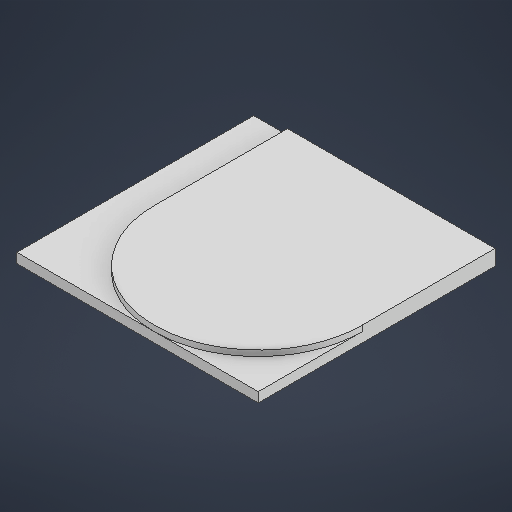
# Autodesk Inventor part: klapka
Saved by Autodesk Inventor 2026.1 (Build 301233020, 233B)
## iProperties
Created: 2025-08-31
Part Number: klapka
Material: Ogólny
Document SubType Name: Modeling
Designer: Paweł
Density: 1 g/cm^3
Appearance: Domyślna
Author: Paweł
Autodesk Inventor part; units mm, degrees
ref_plane "YZ Plane" through (0, 0, 0) normal (1, 0, 0) x (0, 1, 0)
ref_plane "XZ Plane" through (0, 0, 0) normal (0, 1, 0) x (-1, 0, 0)
ref_plane "XY Plane" through (0, 0, 0) normal (0, 0, 1) x (1, 0, 0)
sketch "Sketch1" plane through (0, 0, 0) normal (0, 0, 1) x (1, 0, 0)
  point P0 (0, 0)
sketch "Sketch2" plane through (0, 0, 0) normal (0, 1, 0) x (-1, 0, 0)
  line L0 (11.1114, 10.1278) -> (-7.2886, 10.1278)
  line L1 (-7.2886, 10.1278) -> (-7.2886, -10.8722)
  line L2 (-7.2886, -10.8722) -> (11.1114, -10.8722)
  line L3 (11.1114, -10.8722) -> (11.1114, 10.1278)
  point P0 (0, 0)
  dimension "d0" = 21
  dimension "d1" = 18.4
  constraints: 8 end point, 2 parallel, 1 horizontal, 1 perpendicular
  measures "d0" distance of L2.end L0.start
  measures "d1" distance of L0.start L0.end
extrude "Extrusion1" add sketch "Sketch2" along normal blind 0.5
sketch "Sketch3" plane through (0, 0.5, 0) normal (0, 1, 0) x (1, 0, 0)
  circle A0 centre (-1.9114, -0.9278) radius 9.2
  line L0 (-11.1114, -10.1278) -> (7.2886, -10.1278) projected
  line L1 (7.2886, -10.1278) -> (7.2886, 10.8722) projected
  line L2 (7.2886, -10.1278) -> (7.2886, 10.8722) projected
  line L3 (7.2886, 10.8722) -> (-11.1114, 10.8722) projected
  line L4 (-11.1114, 10.8722) -> (-11.1114, -10.1278) projected
  line L5 (-11.1114, -10.1278) -> (7.2886, -10.1278) projected
  point P0 (0, 0)
  point P1 (-11.1114, -0.9278)
  point P2 (7.2886, -0.9278)
  dimension "d4" = 18.4
  constraints: 2 tangent, 1 centre point
  measures "d4" diameter of A0
extrude "Extrusion2" add sketch "Sketch3" along normal blind 0.5 contours A0 | A0 L4 L3 L1
sketch "Sketch6" plane through (-11.1114, 0, -10.8722) normal (-1, 0, 0) x (0, 0, 1)
  line L0 (0, 0) -> (21, 0) projected
  line L1 (21, 0) -> (21, 0.5) projected
  line L2 (11.8, 0.5) -> (21, 0.5) projected
  line L3 (11.8, 0.5) -> (11.8, 1) projected
  line L4 (0, 1) -> (11.8, 1) projected
  line L5 (0, 0) -> (0, 1) projected
  line L6 (11.8, 0.5) -> (0, 0.5)
  point P0 (10.8722, 0)
  constraints: 2 end point, 1 midpoint
extrude "Extrusion4" add sketch "Sketch6" along normal blind 3 contours L5 L6 L2 L1 L0
sketch "Sketch7" plane through (-14.1114, 0, -10.8722) normal (-1, 0, 0) x (0, 0, 1)
  line L0 (0, 0) -> (0, 1) projected
  line L1 (0, 0.5) -> (0, -0.366)
  line L2 (0, -0.366) -> (21, -0.366)
  line L3 (0, 0) -> (21, 0) projected
  line L4 (21, -0.366) -> (21, 0)
  point P0 (10.8722, 0)
  dimension "d11" = 0.866
  constraints: 6 end point, 2 perpendicular, 1 collinear, 1 midpoint
  measures "d11" distance of L1.start L1.end
extrude "Extrusion5" add sketch "Sketch7" against normal up to surface (21.4 mm away)
body "Solid1"
